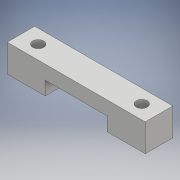
# Autodesk Inventor part: encoder_mounting_clamp
Saved by Autodesk Inventor 2017 (Build 210142000, 142)
## iProperties
Created: 2017-10-30
Part Number: encoder_mounting_clamp
Material: Generic
Document SubType Name: Modeling
Designer: Thoma
Density: 1 g/cm^3
Appearance: Default
Author: Thoma
Autodesk Inventor part; units mm, degrees
ref_plane "YZ Plane" through (0, 0, 0) normal (1, 0, 0) x (0, 1, 0)
ref_plane "XZ Plane" through (0, 0, 0) normal (0, 1, 0) x (-1, 0, 0)
ref_plane "XY Plane" through (0, 0, 0) normal (0, 0, 1) x (1, 0, 0)
sketch "Sketch1" plane through (0, 0, 0) normal (0, 0, 1) x (1, 0, 0)
  line L0 (0, 0) -> (20, 0)
  line L1 (20, 0) -> (20, 4)
  line L2 (20, 4) -> (0, 4)
  line L3 (0, 4) -> (0, 0)
  dimension "d0" = 20
  dimension "d1" = 4
  constraints: 8 end point, 2 parallel, 1 horizontal, 1 perpendicular
  measures "d0" distance of L2.end L1.end
  measures "d1" distance of L1.end L0.end
extrude "Extrusion1" add sketch "Sketch1" along normal blind 4
sketch "Sketch2" plane through (0, 0, 0) normal (0, -1, 0) x (1, 0, 0)
  line L0 (5.5, 0) -> (14.5, 0)
  line L1 (14.5, 0) -> (14.5, 2)
  line L2 (14.5, 2) -> (5.5, 2)
  line L3 (5.5, 2) -> (5.5, 0)
  line L4 (0, 0) -> (20, 0) construction
  line L5 (10, 0) -> (10, 4) construction
  line L6 (0, 4) -> (20, 4) construction
  dimension "d4" = 9
  dimension "d5" = 2
  constraints: 10 end point, 2 midpoint, 2 parallel, 1 horizontal, 1 perpendicular, 1 other
  measures "d4" distance of L2.end L1.end
  measures "d5" distance of L1.end L0.end
extrude "Extrusion2" cut sketch "Sketch2" against normal blind 4
sketch "Sketch3" plane through (0, 0, 4) normal (0, 0, 1) x (1, 0, 0)
  line L0 (0, 2) -> (20, 2) construction
  line L1 (20, 0) -> (20, 4) construction
  line L2 (14.5, 4) -> (5.5, 4) construction
  line L3 (10, 4) -> (10, 0) construction
  line L4 (5.5, 0) -> (14.5, 0) construction
  point P0 (0, 0)
  point P1 (2.5, 2)
  point P2 (17.5, 2)
  dimension "d8" = 15
  constraints: 4 end point, 3 midpoint, 1 point on line, 1 symmetric about line
  measures "d8" distance of point (2.5, 2) point (17.5, 2)
hole "Hole1" at (2.5, 2, 4) at (17.5, 2, 4) direction (0, 0, -1) diameter 1.6 end through all
body "Solid1"
